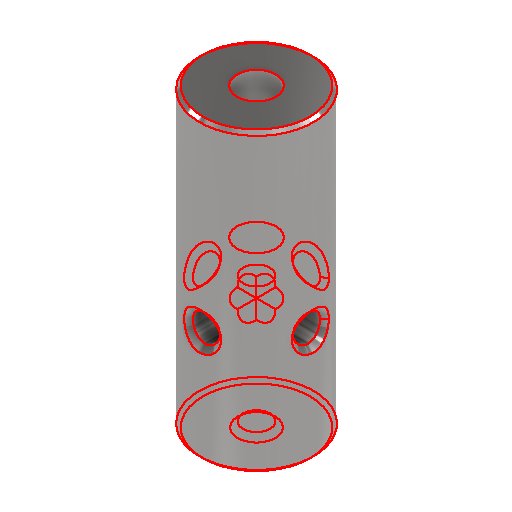
# Autodesk Inventor part: 3DP_PLA_4mm_Adapter__prototype
Saved by Autodesk Inventor 2026.1 (Build 301233000, 233)
## iProperties
Created: 2025-04-04
Part Number: 3DP_PLA_4mm_Adapter__prototype
Material: Generic
Document SubType Name: Modeling
Designer: Andrzej
Density: 1 g/cm^3
Appearance: Stal — polerowana
Author: Andrzej
Autodesk Inventor part; units mm, degrees
ref_plane "YZ Plane" through (0, 0, 0) normal (1, 0, 0) x (0, 1, 0)
ref_plane "XZ Plane" through (0, 0, 0) normal (0, 1, 0) x (-1, 0, 0)
ref_plane "XY Plane" through (0, 0, 0) normal (0, 0, 1) x (1, 0, 0)
sketch "Szkic1" plane through (0, 0, 0) normal (0, 1, 0) x (-1, 0, 0)
  circle A0 centre (0, 0) radius 8.65
  dimension "d0" = 17.3
  constraints: 1 centre point, 1 coincident
  measures "d0" diameter of A0
extrude "Wyciągnięcie proste1" add sketch "Szkic1" along normal blind 45
sketch "Szkic2" plane through (0, 45, 0) normal (0, 1, 0) x (1, 0, 0)
  point P0 (0, 0)
  point P1 (0, 0)
  constraints: 1 coincident
hole "Otwór1" at (0, 45, 0) direction (0, -1, 0) diameter 5.9 depth 20 tip angle 118
sketch "Szkic3" plane through (0, 0, 0) normal (0, -1, 0) x (1, 0, 0)
  point P0 (0, 0)
  point P1 (0, 0)
  constraints: 1 coincident
hole "Otwór2" at (0, 0, 0) direction (0, 1, 0) diameter 4.1 depth 20 tip angle 118
sketch "Szkic4" plane through (0, 0, 0) normal (0, 0, 1) x (1, 0, 0)
  circle A0 centre (0, 17) radius 2.05
  point P0 (0, 0)
  dimension "d17" = 17
  dimension "d18" = 4.1
  constraints: 1 centre point, 1 coincident, 1 vertical alignment
  measures "d17" distance of point (0, 0) point (0, 17)
  measures "d18" diameter of A0
extrude "Wyciągnięcie proste2" cut sketch "Szkic4" along normal through all both and the other way through all
pattern_circular "Szyk kołowy1" count 2 over 90 about axis through (0, -10, 0) along (0, 1, 0) of "Wyciągnięcie proste2"
chamfer "Faza1" distance 0.5 angle 45 2 edges at (8.65, 45, 0) (8.65, 0, 0)
chamfer "Faza2" distance 0.8 angle 45 7 edges at (0, 0, 2.05) (-8.5095, 15.6615, -1.5527) (-8.5094, 18.3376, -1.5535) (-8.4036, 17.0002, 2.05) (8.4036, 17.0023, 2.05) (-2.05, 17.0105, 8.4036) (-2.05, 17.0105, -8.4036)
